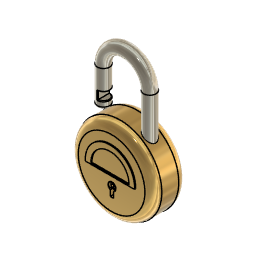
Lock_Model (Autodesk Fusion 360 design; units mm, degrees)
Autodesk Fusion 360 part; units mm, degrees
note: some values were not read from the file. Chosen so that the rebuilt part matches the saved one: which face or edge a step refers to.
sketch "Sketch1" plane through (0, 0, 0) normal (0, 1, 0) x (1, 0, 0)
sketch "Sketch2" plane through (0, 0, 0) normal (0, 1, 0) x (1, 0, 0)
sketch "Sketch3" plane through (0, 0, 0) normal (0, 1, 0) x (1, 0, 0)
  circle A0 centre (90.8394, -2.3155) radius 24.7054
  line L0 (92, 6.5608) -> (92, 10)
  line L1 (92, 10) -> (90.0615, 10)
  line L2 (90.0615, 10) -> (90.0615, 6.5608)
  line L3 (90.4643, 2.6624) -> (90.4643, 4.1624)
  line L4 (90.4643, 4.1624) -> (90.4643, 2.6624)
  line L5 (92.0727, 2.6624) -> (92.0727, 5.6624)
  arc A1 (92.8139, 2.9327) -> (92.0727, 5.6624) centre (91.0514, 3.9196) ccw
  line L6 (92.0727, 2.6624) -> (90.4643, 2.6624)
  arc A2 (90.4643, 4.1624) -> (90.2999, 5.1624) centre (90.2837, 4.6462) ccw
  arc A3 (90.0687, 5.7436) -> (90.2999, 5.1624) centre (90.3106, 5.5032) ccw
  arc A4 (90.0687, 5.7436) -> (88.9128, 3.6415) centre (90.5346, 4.1186) ccw
  arc A5 (90.0615, 6.5608) -> (92, 6.6052) centre (91.0791, 4.4747) ccw
  constraint vertical L0
  constraint horizontal L1
  constraint vertical L2
  constraint vertical L3
  constraint parallel L4 L5
  constraint coincident A1.start A5
  constraint perpendicular L3 L6
  constraint tangent A2 A3
  constraint coincident A4.end A5
  constraint coincident L0 A5.end
extrude "Extrude1" add sketch "Sketch3" along normal blind 20 contours A0 | L0 L1 L2 L3 L4 L5 A1 L6 A2 A3 A4 A5 | L3 L4 L5 A1 L6 A2 A3 A4 A5 makes body 1
fillet "Fillet1" radius 5 1 edges at (67.8058, 0, 11.2494) on bodies 1
fillet "Fillet2" radius 5 1 edges at (67.8058, 20, 11.2494) on bodies 1
sketch "Sketch4" plane through (0, 0, 0) normal (0, 1, 0) x (1, 0, 0)
extrude "Extrude2" cut sketch "Sketch3" along normal blind 10 contours L0 L1 L2 L3 L4 L5 A1 L6 A2 A3 A4 A5 bodies 1
sketch "Sketch5" plane through (0, 0, 0) normal (0, 1, 0) x (1, 0, 0)
sketch "Sketch6" plane through (0, 0, 0) normal (0, 1, 0) x (1, 0, 0)
sketch "Sketch7" plane through (0, 0, 0) normal (0, 1, 0) x (1, 0, 0)
extrude "Extrude3" add sketch "Sketch3" along normal blind 10 contours L0 L1 L2 L3 L4 L5 A1 L6 A2 A3 A4 A5 bodies 1
extrude "Extrude4" cut sketch "Sketch3" along normal blind 10 contours L0 L1 L2 L3 L4 L5 A1 L6 A2 A3 A4 A5 bodies 1
sketch "Sketch8" plane through (0, 0, 0) normal (0, 0, 1) x (1, 0, 0)
sketch "Sketch9" plane through (0, 0, 0) normal (0, 1, 0) x (1, 0, 0)
sketch "Sketch10" plane through (0, 0, 0) normal (0, 1, 0) x (1, 0, 0)
sketch "Sketch11" plane through (0, 0, 0) normal (0, 1, 0) x (1, 0, 0)
  line L0 (67.4023, -40.881) -> (67.4023, -70)
  line L1 (105, -70) -> (105, -30)
  arc A0 (67.4023, -70) -> (105, -70) centre (86.2012, -70) ccw
  constraint vertical L0
  constraint tangent L1 A0
pipe "Pipe1" add diameter 10 path "Sketch11" along L0 A0 L1 separate body makes body 2
fillet "Fillet3" radius 2 1 edges at (62.7407, -1.8081, 40.881) on bodies 2
fillet "Fillet4" radius 2 1 edges at (109.6616, -1.8081, 30) on bodies 2
sketch "Sketch12" plane through (0, 0, 0) normal (0, 1, 0) x (1, 0, 0)
  line L0 (67.6466, -53.3473) -> (75.2087, -53.3473)
  line L1 (75.2087, -53.3473) -> (75.2087, -47.0226)
  line L2 (75.2087, -47.0226) -> (67.6466, -47.0226)
  line L3 (67.6466, -47.0226) -> (67.6466, -53.3473)
  constraint horizontal L0
  constraint vertical L1
  constraint horizontal L2
  constraint vertical L3
extrude "Extrude5" cut sketch "Sketch12" along normal mid plane 60 bodies 2
fillet "Fillet5" radius 0.5 6 edges at (71.0232, 3.4481, 47.0226) (67.6466, 4.994, 50.185) (71.0232, 3.4481, 53.3473) (71.0232, -3.4481, 53.3473) (67.6466, -4.994, 50.185) (71.0232, -3.4481, 47.0226) on bodies 2
scale "Scale1" factor 0.883045 about (62.4023, 0, 70) bodies 2
scale "Scale2" factor 0.824568 about (62.4023, 0, 70) bodies 2
ref_plane "WorkPlane1" through (90.8394, 11.0475, 27.021) normal (0, 0, 1) x (-1, 0, 0)
sketch "Sketch13" plane through (0, 0, 27.021) normal (0, 0, 1) x (1, 0, 0)
  circle A0 centre (103.5704, 9.8579) radius 3.5
  dimension "d28" = 7
  measures "d28" diameter of A0
extrude "Extrude6" cut sketch "Sketch13" against normal blind 10 bodies 1
move_body "Move1" bodies 2 to x (1, 0, 0) y (0, 1, 0) z (0, 0, 1) at (10.1514, 9.8579, -23.8538)
sketch "Sketch14" plane through (0, 0, 0) normal (0, -1, 0) x (1, 0, 0)
  arc A0 (92.0727, -5.6624) -> (92.8139, -2.9327) centre (91.0514, -3.9196) ccw
  arc A1 (92, -6.6052) -> (92.8139, -2.9327) centre (91.0791, -4.4747) ccw
  line L0 (92, -6.6052) -> (92, -10)
  line L1 (92, -10) -> (90.0615, -10)
  line L2 (90.0615, -10) -> (90.0615, -6.5608)
  arc A2 (88.9128, -3.6415) -> (90.0615, -6.5608) centre (91.0791, -4.4747) ccw
  arc A3 (88.9128, -3.6415) -> (90.0687, -5.7436) centre (90.5346, -4.1186) ccw
  arc A4 (90.2999, -5.1624) -> (90.0687, -5.7436) centre (90.3106, -5.5032) ccw
  arc A5 (90.2999, -5.1624) -> (90.4643, -4.1624) centre (90.2837, -4.6462) ccw
  line L3 (90.4643, -4.1624) -> (90.4643, -2.6624)
  line L4 (90.4643, -2.6624) -> (92.0727, -2.6624)
  line L5 (92.0727, -2.6624) -> (92.0727, -5.6624)
  circle A6 centre (90.8394, 2.3155) radius 19.7054
  arc A7 (92.8139, -2.9327) -> (88.9128, -3.6415) centre (91.0415, -4.2676) ccw
  arc A8 (93.0696, -4.0027) -> (89.1978, -5.1533) centre (91.0415, -4.2676) ccw
  arc A9 (88.9128, -3.6415) -> (89.1978, -5.1533) centre (90.4003, -4.1439) ccw
  arc A10 (93.0696, -4.0027) -> (92.8139, -2.9327) centre (91.0514, -3.9196) ccw
  arc A11 (92.8139, -2.9327) -> (88.9128, -3.6415) centre (91.0415, -4.2676) ccw
  constraint tangent A3 A7
  constraint coincident A0.end A1.end
  constraint coincident A2.start A3.start
  constraint concentric A7 A8
  constraint coincident A3 A8.end
  constraint coincident A0 A8.start
  constraint tangent A3 A11
extrude "Extrude7" cut sketch "Sketch14" against normal blind 10 contours A0 A3 A7 A8 A10 A11 bodies 1
sketch "Sketch15" plane through (0, 0, 0) normal (0, -1, 0) x (1, 0, 0)
  circle A0 centre (90.8394, 2.3155) radius 19.7054
  arc A1 (92.8139, -2.9327) -> (88.9128, -3.6415) centre (91.0415, -4.2676) ccw
  arc A2 (92, -6.6052) -> (92.8139, -2.9327) centre (91.0791, -4.4747) ccw
  line L0 (92, -6.6052) -> (92, -10)
  line L1 (92, -10) -> (90.0615, -10)
  line L2 (90.0615, -10) -> (90.0615, -6.5608)
  arc A3 (88.9128, -3.6415) -> (90.0615, -6.5608) centre (91.0791, -4.4747) ccw
  line L3 (75.9273, 1.3266) -> (105, 1.3266)
  arc A4 (105, 1.3266) -> (75.9273, 1.3266) centre (90.4637, 2.304) ccw
  line L4 (79.2023, 2) -> (101.725, 2)
  arc A5 (101.725, 2) -> (79.2023, 2) centre (90.4637, 2.304) ccw
  constraint horizontal L3
  constraint parallel L3 L4
extrude "Extrude8" add sketch "Sketch15" along normal blind 0.6 contours L3 A4 bodies 1
